Screen (Autodesk Fusion 360 design; units mm, degrees)
Autodesk Fusion 360 part; units mm, degrees
note: some values were not read from the file. Set by a fixed rule: which sketch regions a step uses.
sketch "Sketch1" plane through (0, 0, 0) normal (0, 0, 1) x (1, 0, 0)
  line L0 (18, 0) -> (170, 0)
  line L1 (188, 18) -> (188, 150)
  line L2 (188, 150) -> (0, 150)
  line L3 (0, 150) -> (0, 18)
  arc A0 (170, 0) -> (188, 18) centre (170, 18) ccw
  arc A1 (0, 18) -> (18, 0) centre (18, 18) ccw
  line L4 (186, 20) -> (186, 148)
  line L5 (186, 148) -> (2, 148)
  line L6 (2, 148) -> (2, 20)
  line L7 (21.5, 116) -> (166.5, 116)
  line L8 (171.5, 111) -> (171.5, 36)
  line L9 (166.5, 31) -> (21.5, 31)
  line L10 (16.5, 36) -> (16.5, 111)
  arc A2 (166.5, 31) -> (171.5, 36) centre (166.5, 36) ccw
  arc A3 (171.5, 111) -> (166.5, 116) centre (166.5, 111) ccw
  arc A4 (21.5, 116) -> (16.5, 111) centre (21.5, 111) ccw
  arc A5 (16.5, 36) -> (21.5, 31) centre (21.5, 36) ccw
  arc A6 (181.5, 111) -> (166.5, 126) centre (166.5, 111) ccw
  line L11 (21.5, 126) -> (166.5, 126)
  arc A7 (21.5, 126) -> (6.5, 111) centre (21.5, 111) ccw
  line L12 (6.5, 36) -> (6.5, 111)
  arc A8 (6.5, 36) -> (21.5, 21) centre (21.5, 36) ccw
  line L13 (166.5, 21) -> (21.5, 21)
  arc A9 (166.5, 21) -> (181.5, 36) centre (166.5, 36) ccw
  line L14 (181.5, 111) -> (181.5, 36)
  arc A10 (2, 20) -> (18, 4) centre (18, 20) ccw
  line L15 (18, 4) -> (170, 4)
  arc A11 (170, 4) -> (186, 20) centre (170, 20) ccw
  line L16 (321.5, 126) -> (466.5, 126)
  arc A12 (481.5, 111) -> (466.5, 126) centre (466.5, 111) ccw
  line L17 (481.5, 111) -> (481.5, 36)
  arc A13 (466.5, 21) -> (481.5, 36) centre (466.5, 36) ccw
  line L18 (466.5, 21) -> (321.5, 21)
  arc A14 (306.5, 36) -> (321.5, 21) centre (321.5, 36) ccw
  line L19 (306.5, 36) -> (306.5, 111)
  arc A15 (321.5, 126) -> (306.5, 111) centre (321.5, 111) ccw
  arc A16 (485.5, 111) -> (466.5, 130) centre (466.5, 111) ccw
  line L20 (321.5, 130) -> (466.5, 130)
  arc A17 (321.5, 130) -> (302.5, 111) centre (321.5, 111) ccw
  line L21 (302.5, 36) -> (302.5, 111)
  arc A18 (302.5, 36) -> (321.5, 17) centre (321.5, 36) ccw
  line L22 (466.5, 17) -> (321.5, 17)
  arc A19 (466.5, 17) -> (485.5, 36) centre (466.5, 36) ccw
  line L23 (485.5, 111) -> (485.5, 36)
  point P0 (188, 0)
  point P1 (16.5, 116)
  point P2 (171.5, 116)
  point P3 (16.5, 31)
  dimension "d1" = 188
  dimension "d2" = 150
  dimension "d3" = 18
  dimension "d5" = 155
  dimension "d6" = 85
  dimension "d7" = 14.5
  dimension "d9" = 5
  dimension "d10" = -10
  dimension "d41" = -4
  constraint horizontal L0
  constraint vertical L1
  constraint horizontal L2
  constraint vertical L3
  constraint coincident P0 L0
  constraint coincident P0 L1
  constraint tangent L0 A0
  constraint tangent L1 A0
  constraint coincident origin L0
  constraint coincident origin L3
  constraint tangent L0 A1
  constraint tangent L3 A1
  constraint equal A0 A1
  constraint horizontal L7
  constraint vertical L8
  constraint horizontal L9
  constraint vertical L10
  constraint tangent L8 A2
  constraint tangent L9 A2
  constraint coincident P2 L7
  constraint coincident P2 L8
  constraint tangent L7 A3
  constraint tangent L8 A3
  constraint equal A2 A3
  constraint coincident P1 L7
  constraint coincident P1 L10
  constraint tangent L7 A4
  constraint tangent L10 A4
  constraint equal A2 A4
  constraint coincident P3 L9
  constraint coincident P3 L10
  constraint tangent L9 A5
  constraint tangent L10 A5
  constraint equal A2 A5
  constraint parallel L1 L4
  constraint parallel L2 L5
  constraint parallel L3 L6
  measures "d1" distance of origin P0
  measures "d2" distance of origin L2.end
  measures "d3" radius of A0
  measures "d5" distance of P1 P2
  measures "d6" distance of P1 P3
  measures "d7" distance of L6 L10
  measures "d9" radius of A2
  measures "d10" distance of A3
extrude "Extrude7" add sketch "Sketch1" along normal blind 2 contours A16 L20 A17 L21 A18 L22 A19 L23 makes body 1
extrude "Extrude1" add sketch "Sketch1" along normal blind 2 separate body contours L0 L1 L2 L3 A0 A1 makes body 2
extrude "Extrude2" add sketch "Sketch1" along normal blind 10 contours L4 L5 L6 A10 L15 A11 | L7 L8 L9 L10 A2 A3 A4 A5 | A6 L11 A7 L12 A8 L13 A9 L14 bodies 2
extrude "Extrude3" cut sketch "Sketch1" along normal blind 10 draft -45 contours L7 L8 L9 L10 A2 A3 A4 A5 | A6 L11 A7 L12 A8 L13 A9 L14 bodies 2
sketch "Sketch3" plane through (0, 0, 10) normal (0, 0, 1) x (-1, 0, 0)
  line L0 (-21.5, -116) -> (-166.5, -116)
  arc A0 (-171.5, -111) -> (-166.5, -116) centre (-166.5, -111) ccw
  line L1 (-171.5, -111) -> (-171.5, -36)
  arc A1 (-166.5, -31) -> (-171.5, -36) centre (-166.5, -36) ccw
  line L2 (-166.5, -31) -> (-21.5, -31)
  arc A2 (-16.5, -36) -> (-21.5, -31) centre (-21.5, -36) ccw
  line L3 (-16.5, -36) -> (-16.5, -111)
  arc A3 (-21.5, -116) -> (-16.5, -111) centre (-21.5, -111) ccw
  line L4 (-186, -20) -> (-186, -148)
  line L5 (-186, -148) -> (-2, -148)
  line L6 (-2, -148) -> (-2, -20)
  line L7 (-16.4268, -115.8738) -> (-171.4268, -115.8738)
  line L8 (-171.4268, -115.8738) -> (-171.4268, -30.8738)
  line L9 (-171.4268, -30.8738) -> (-16.4268, -30.8738)
  line L10 (-16.4268, -30.8738) -> (-16.4268, -115.8738)
  line L11 (-21.5, -116) -> (-166.5, -116)
  line L12 (-9.9268, -122.2738) -> (-174.9268, -122.2738)
  line L13 (-174.9268, -122.2738) -> (-174.9268, -21.8738)
  line L14 (-174.9268, -21.8738) -> (-9.9268, -21.8738)
  line L15 (-9.9268, -21.8738) -> (-9.9268, -122.2738)
  line L16 (-179.9268, -16.8738) -> (-4.9268, -16.8738)
  line L17 (-4.9268, -16.8738) -> (-4.9268, -127.2738)
  line L18 (-4.9268, -127.2738) -> (-179.9268, -127.2738)
  line L19 (-179.9268, -127.2738) -> (-179.9268, -16.8738)
  line L20 (-92.4268, -16.8738) -> (-92.4268, -21.8738) construction
  line L21 (-67.4268, -21.8738) -> (-67.4268, -16.8738)
  line L22 (-117.4268, -21.8738) -> (-117.4268, -16.8738)
  arc A4 (-170, -4) -> (-186, -20) centre (-170, -20) ccw
  arc A5 (-2, -20) -> (-18, -4) centre (-18, -20) ccw
  line L23 (-18, -4) -> (-170, -4)
  dimension "d17" = 155
  dimension "d18" = 85
  dimension "d20" = 165
  dimension "d21" = 100.4
  dimension "d22" = 6.5
  dimension "d23" = 6.4
  dimension "d24" = -5
  dimension "d25" = 25
  dimension "d26" = 25
  constraint horizontal L7
  constraint vertical L8
  constraint horizontal L9
  constraint vertical L10
  constraint horizontal L12
  constraint vertical L13
  constraint horizontal L14
  constraint vertical L15
  constraint midpoint L16 L20.start
  constraint midpoint L14 L20.end
  constraint coincident L14 L21.start
  constraint coincident L16 L21.end
  constraint perpendicular L16 L21
  constraint coincident L14 L22.start
  constraint coincident L16 L22.end
  constraint perpendicular L16 L22
  measures "d17" distance of L7.start L7.end
  measures "d18" distance of L7.start L9.end
  measures "d20" distance of L12.start L12.end
  measures "d21" distance of L12.start L14.end
  measures "d22" distance of L10 L15
  measures "d23" distance of L7 L12
  measures "d25" distance of L20 L22
  measures "d26" distance of L20 L21
extrude "Extrude4" add sketch "Sketch3" along normal blind 10 contours L12 L13 L14 L15 L16 L17 L18 L19 L21 L22 bodies 2
sketch "Sketch4" plane through (179.9268, 0, 0) normal (1, 0, 0) x (0, 1, 0)
  line L0 (16.8738, 10) -> (127.2738, 10)
  line L1 (127.2738, 10) -> (127.2738, 20)
  line L2 (127.2738, 20) -> (16.8738, 20)
  line L3 (16.8738, 20) -> (16.8738, 10)
  line L4 (62.0738, 15) -> (82.0738, 15)
  line L5 (82.0738, 15) -> (82.0738, 13)
  line L6 (82.0738, 13) -> (62.0738, 13)
  line L7 (62.0738, 13) -> (62.0738, 15)
  dimension "d29" = 20
  dimension "d30" = 2
  dimension "d31" = 3
  dimension "d32" = 45.2
  constraint horizontal L4
  constraint vertical L5
  constraint horizontal L6
  constraint vertical L7
  measures "d29" distance of L4.start L4.end
  measures "d30" distance of L4.start L6.end
  measures "d31" distance of L0 L6
  measures "d32" distance of L1 L5
extrude "Extrude5" cut sketch "Sketch4" against normal blind 200 contours L4 L5 L6 L7 bodies 2
sketch "Sketch5" plane through (0, 127.2738, 0) normal (0, 1, 0) x (-1, 0, 0)
  line L0 (-179.9268, 10) -> (-4.9268, 10)
  line L1 (-4.9268, 10) -> (-4.9268, 20)
  line L2 (-4.9268, 20) -> (-179.9268, 20)
  line L3 (-179.9268, 20) -> (-179.9268, 10)
  line L4 (-102.4268, 15) -> (-82.4268, 15)
  line L5 (-82.4268, 15) -> (-82.4268, 13)
  line L6 (-82.4268, 13) -> (-102.4268, 13)
  line L7 (-102.4268, 13) -> (-102.4268, 15)
  dimension "d35" = 20
  dimension "d36" = 2
  dimension "d37" = 3
  dimension "d38" = 77.5
  constraint horizontal L4
  constraint vertical L5
  constraint horizontal L6
  constraint vertical L7
  measures "d35" distance of L4.start L4.end
  measures "d36" distance of L4.start L6.end
  measures "d37" distance of L0 L6
  measures "d38" distance of L1 L4.end
extrude "Extrude6" cut sketch "Sketch5" against normal blind 10 contours L4 L5 L6 L7 bodies 2
fillet "Fillet1" radius 2 8 edges at (485.5, 73.5, 2) (479.935, 124.435, 2) (394, 130, 2) (308.065, 124.435, 2) (302.5, 73.5, 2) (308.065, 22.565, 2) (394, 17, 2) (479.935, 22.565, 2) on bodies 1
fillet "Fillet2" radius 2 8 edges at (481.5, 73.5, 2) (477.1066, 25.3934, 2) (394, 21, 2) (310.8934, 25.3934, 2) (306.5, 73.5, 2) (310.8934, 121.6066, 2) (394, 126, 2) (477.1066, 121.6066, 2) on bodies 1
